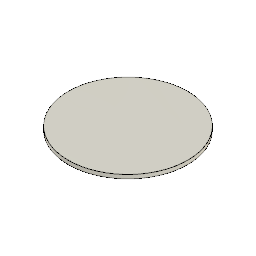
Flat_Disk_v1 (Autodesk Fusion 360 design; units mm, degrees)
Autodesk Fusion 360 part; units mm, degrees
cylinder "CylinderPrimitive1" add diameter 76.2 height 2.54 placed x (1, 0, 0) y (0, 1, 0) z (0, 0, 1) at (40.64, 38.1, 0) in component "Disk"
component "Disk" placed x (1, 0, 0) y (0, 1, 0) z (0, 0, 1) at (0, 0, 0)
component "Component" placed x (1, 0, 0) y (0, 1, 0) z (0, 0, 1) at (0, 0, 0)
